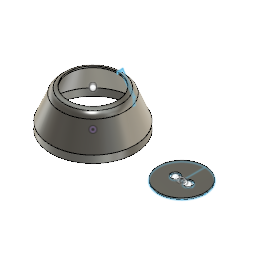
case (Autodesk Fusion 360 design; units mm, degrees)
Autodesk Fusion 360 part; units mm, degrees
sketch "Sketch1" plane through (0, 0, 0) normal (1, 0, 0) x (0, 1, 0)
  line L0 (0, 76) -> (0, 73)
  line L1 (85, 0) -> (85, 15)
  line L2 (85, 15) -> (60, 76)
  line L3 (60, 76) -> (50, 76)
  line L4 (50, 76) -> (50, 73)
  line L5 (50, 73) -> (57, 73)
  line L6 (85, 0) -> (82, 0)
  line L7 (82, 0) -> (82, 15)
  line L8 (82, 15) -> (57, 73)
  dimension "d3" = 76
  dimension "d7" = 3
  dimension "d18" = 10
  dimension "d20" = 7
  dimension "d21" = 3
  dimension "d23" = 15
  dimension "d24" = 85
  dimension "d26" = 3
  constraint perpendicular L4 L5
  constraint perpendicular L6 L7
  measures "d3" distance of origin L0.start
  measures "d7" distance of L0.start L0.end
  measures "d18" distance of L2.end L3.end
  measures "d20" distance of L4.end L5.end
  measures "d21" distance of L1.start L6.end
  measures "d23" distance of L6.end L7.end
  measures "d24" distance of origin L1.start
  measures "d26" distance of L3.end L4.end
revolve "Revolve1" add sketch "Sketch1" angle 360 about axis through (0, 0, 1.75) along (0, 0, 1) makes body 1
fillet "Fillet1" radius 20 1 edges at (-55.9396, 21.6969, 76) on bodies 1
sketch "Sketch2" plane through (0, 0, 0) normal (0, 0, 1) x (1, 0, 0)
  circle A0 centre (180, 0) radius 47
  line L0 (180, 0) -> (180, 47)
  line L1 (180, 0) -> (175.5, 0)
  circle A1 centre (167, 0) radius 8.5
  circle A2 centre (193, 0) radius 8.5
  line L2 (180, 0) -> (184.5, 0)
  dimension "d30" = 94
  dimension "d31" = 47
  dimension "d32" = 4.5
  dimension "d33" = 17
  dimension "d34" = 17
  dimension "d35" = 4.5
  constraint coincident A0.centre L0.start
  constraint coincident A0 L0.end
  constraint vertical L0
  constraint perpendicular L0 L1
  constraint perpendicular L0 L2
  measures "d30" diameter of A0
  measures "d31" distance of A0.centre L0.end
  measures "d32" distance of A0.centre L1.end
  measures "d33" diameter of A1
  measures "d34" diameter of A2
  measures "d35" distance of A0.centre L2.end
extrude "Extrude1" add sketch "Sketch2" along normal blind 3 separate body makes body 2
